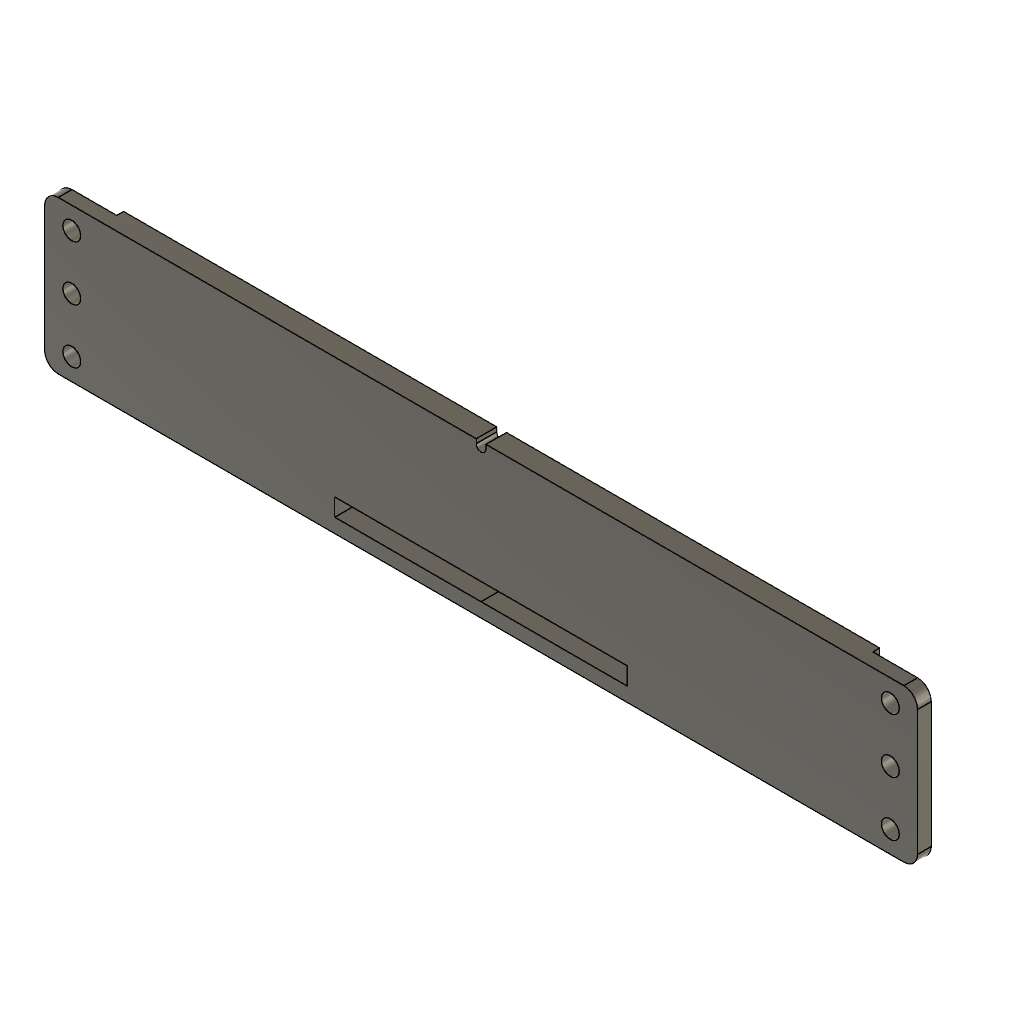
elgato-streamdeck-neo-10-inch-rack-mount (Autodesk Fusion 360 design; units mm, degrees)
Autodesk Fusion 360 part; units mm, degrees
sketch "Sketch1" plane through (0, 0, 0) normal (0, 1, 0) x (1, 0, 0)
  line L0 (127, -22.25) -> (-127, -22.25)
  line L1 (-127, -22.25) -> (-127, 22.25)
  line L2 (-127, 22.25) -> (127, 22.25)
  line L3 (127, 22.25) -> (127, -22.25)
  line L4 (127, -22.25) -> (-127, 22.25) construction
  line L5 (-127, -22.25) -> (127, 22.25) construction
  line L6 (-127, -22.25) -> (-111.125, -22.25) construction
  line L7 (-111.125, -22.25) -> (-111.125, 22.25) construction
  line L8 (-111.125, 22.25) -> (-127, 22.25) construction
  line L9 (-127, 22.25) -> (-127, -22.25) construction
  line L10 (-127, -22.25) -> (-110, -22.25)
  line L11 (-110, -22.25) -> (-110, 22.25)
  line L12 (-110, 22.25) -> (-127, 22.25)
  line L13 (-127, 22.25) -> (-127, -22.25)
  line L14 (-127, -22.25) -> (-111.125, 22.25) construction
  circle A0 centre (-119.0625, 0) radius 2.6
  circle A1 centre (-119.0625, 0) radius 2.5 construction
  circle A2 centre (-119.0625, -15.875) radius 2.6
  circle A3 centre (-119.0625, 15.875) radius 2.6
  line L15 (0, -22.25) -> (0, 22.25) construction
  circle A4 centre (119.0625, -15.875) radius 2.6
  line L16 (127, 22.25) -> (127, -22.25)
  line L17 (111.125, -22.25) -> (111.125, 22.25) construction
  line L18 (127, -22.25) -> (111.125, 22.25) construction
  line L19 (127, -22.25) -> (127, 22.25)
  line L20 (110, -22.25) -> (110, 22.25)
  line L21 (127, -22.25) -> (111.125, -22.25) construction
  circle A5 centre (119.0625, 0) radius 2.5 construction
  line L22 (111.125, 22.25) -> (127, 22.25) construction
  circle A6 centre (119.0625, 15.875) radius 2.6
  line L23 (110, 22.25) -> (127, 22.25)
  line L24 (127, 22.25) -> (127, -22.25) construction
  circle A7 centre (119.0625, 0) radius 2.6
  line L25 (127, -22.25) -> (110, -22.25)
  dimension "d1" = 254
  dimension "d2" = 44.5
  dimension "d3" = 15.875
  dimension "d4" = 17
  dimension "d5" = 5.2
  dimension "d9" = 0
  dimension "d10" = 15.875
  dimension "d18" = 15.875
  constraint horizontal L0
  constraint perpendicular L0 L1
  constraint parallel L0 L2
  constraint parallel L1 L3
  constraint coincident L4 origin
  constraint coincident L5 origin
  constraint horizontal L6
  constraint vertical L7
  constraint horizontal L8
  constraint vertical L9
  constraint horizontal L10
  constraint vertical L11
  constraint horizontal L12
  constraint vertical L13
  constraint midpoint L14 A0.centre
  constraint concentric A0 A1
  constraint midpoint L0 L15.start
  constraint midpoint L2 L15.end
  constraint symmetric L0.end L15 L0.start
  constraint symmetric L1.end L15 L2.end
  constraint symmetric L6.end L15 L17.start
  constraint symmetric L7.end L15 L17.end
  constraint symmetric L10.end L15 L20.start
  constraint symmetric L11.end L15 L20.end
  constraint symmetric A0 L15 A7
  constraint symmetric A1 L15 A5
  constraint symmetric A2 L15 A4
  constraint symmetric A3 L15 A6
  measures "d1" distance of L1.end L2.end
  measures "d2" distance of L0.end L1.end
  measures "d3" distance of L0.end L6.end
  measures "d4" distance of L0.end L10.end
  measures "d5" diameter of A0
  measures "d18" distance of A0.centre A2.centre
extrude "Extrude1" add sketch "Sketch1" along normal blind 4
extrude "Extrude2" add sketch "Sketch1" along normal blind 6 contours L0 L2 L11 L20
fillet "Fillet1" radius 4 4 edges at (127, 2, 22.25) (127, 2, -22.25) (-127, 2, -22.25) (-127, 2, 22.25)
sketch "Sketch2" plane through (0, 0, 0) normal (0, 1, 0) x (1, 0, 0)
  line L0 (0, 13) -> (-42.5625, 13)
  line L1 (-42.5625, 13) -> (-42.5625, 18.0675)
  line L2 (-42.5625, 18.0675) -> (0, 18.0675)
  line L3 (0, 18.0675) -> (0, 13)
  line L4 (0, 13) -> (42.5073, 13)
  line L5 (42.5073, 13) -> (42.5073, 18.0969)
  line L6 (42.5073, 18.0969) -> (0, 18.0969)
  line L7 (0, 18.0969) -> (0, 13)
  constraint horizontal L0
  constraint vertical L1
  constraint horizontal L2
  constraint vertical L3
  constraint horizontal L4
  constraint vertical L5
  constraint horizontal L6
  constraint vertical L7
extrude "Extrude3" cut sketch "Sketch2" along normal blind 460
extrude "Extrude4" cut 1 faces at (-28.375, 4, -18.0675) along direction (0, 0, -1) blind 0.03
sketch "Sketch3" plane through (0, 6, 0) normal (0, 1, 0) x (-1, 0, 0)
  line L0 (0, -18.0975) -> (0, -18.0969)
  line L1 (0, -18.0969) -> (-42.5073, -18.0969)
  line L2 (-42.5073, -18.0969) -> (-42.5073, -13)
  line L3 (-42.5073, -13) -> (42.5625, -13)
  line L4 (42.5625, -13) -> (42.5625, -18.0975)
  line L5 (42.5625, -18.0975) -> (0, -18.0975)
  line L6 (110, 22.25) -> (-110, 22.25)
  line L7 (-110, 22.25) -> (-110, -22.25)
  line L8 (-110, -22.25) -> (110, -22.25)
  line L9 (110, -22.25) -> (110, 22.25)
  line L10 (-45, -10) -> (45, -10)
  line L11 (45, -10) -> (45, -20)
  line L12 (45, -20) -> (-45, -20)
  line L13 (-45, -20) -> (-45, -10)
  constraint horizontal L10
  constraint vertical L11
  constraint horizontal L12
  constraint vertical L13
extrude "Extrude5" add sketch "Sketch3" along normal blind 12 contours L10 L11 L12 L13
sketch "Sketch4" plane through (0, 0, 0) normal (0, -1, 0) x (1, 0, 0)
  arc A0 (-123, 22.25) -> (-127, 18.25) centre (-123, 18.25) ccw
  line L0 (-127, 18.25) -> (-127, -18.25)
  arc A1 (-127, -18.25) -> (-123, -22.25) centre (-123, -18.25) ccw
  line L1 (-123, -22.25) -> (123, -22.25)
  arc A2 (123, -22.25) -> (127, -18.25) centre (123, -18.25) ccw
  line L2 (127, -18.25) -> (127, 18.25)
  arc A3 (127, 18.25) -> (123, 22.25) centre (123, 18.25) ccw
  line L3 (123, 22.25) -> (-123, 22.25)
  circle A4 centre (119.0625, 0) radius 2.6
  circle A5 centre (119.0625, 15.875) radius 2.6
  circle A6 centre (119.0625, -15.875) radius 2.6
  circle A7 centre (-119.0625, 15.875) radius 2.6
  circle A8 centre (-119.0625, -15.875) radius 2.6
  circle A9 centre (-119.0625, 0) radius 2.6
  line L4 (0, -18.0969) -> (0, -18.0975)
  line L5 (0, -18.0975) -> (-42.5625, -18.0975)
  line L6 (-42.5625, -18.0975) -> (-42.5625, -13)
  line L7 (-42.5625, -13) -> (42.5073, -13)
  line L8 (42.5073, -13) -> (42.5073, -18.0969)
  line L9 (42.5073, -18.0969) -> (0, -18.0969)
  circle A10 centre (0, 21) radius 1.4142
  line L10 (-1.4142, 21.0088) -> (-1.4065, 22.25)
  line L11 (1.4142, 21.0088) -> (1.4065, 22.25)
  constraint coincident A10 L10.start
  constraint coincident L3 L10.end
  constraint tangent A10 L10
  constraint coincident A10 L11.start
  constraint coincident L3 L11.end
  constraint tangent A10 L11
extrude "Extrude6" cut sketch "Sketch4" against normal blind 11.5 contours L3 A10 L10 | L3 A10 | L3 A10 L11 picked at (0.2336, 20.1841)
